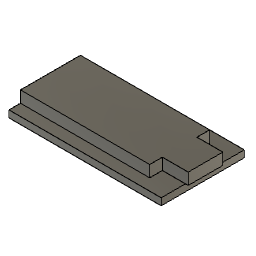
ArduinoProMicro_Pinless (Autodesk Fusion 360 design; units mm, degrees)
Autodesk Fusion 360 part; units mm, degrees
sketch "スケッチ1" plane through (0, 0, 0) normal (0, 0, 1) x (1, 0, 0)
  line L0 (0, 0) -> (33, 0)
  line L1 (33, 0) -> (33, 18)
  line L2 (33, 18) -> (0, 18)
  line L3 (0, 18) -> (0, 0)
  dimension "d1" = 33
  dimension "d2" = 18
  constraint horizontal L0
  constraint vertical L1
  constraint horizontal L2
  constraint vertical L3
  constraint coincident L0.start L3.end
  measures "d1" distance of L0.start L0.end
  measures "d2" distance of L0.start L2.end
extrude "押し出し1" add sketch "スケッチ1" along normal blind 4
sketch "スケッチ2" plane through (0, 0, 4) normal (0, 0, 1) x (-1, 0, 0)
  line L0 (0, -18) -> (0, 0)
  line L1 (0, 0) -> (-33, 0)
  line L2 (-33, 0) -> (-33, -18)
  line L3 (-33, -18) -> (0, -18)
  line L4 (-33, -18) -> (-28, -18)
  line L5 (-28, -18) -> (-28, 0)
  line L6 (-28, 0) -> (-33, 0)
  line L7 (-33, 0) -> (-33, -18)
  line L8 (-28, -12.75) -> (-33, -12.75)
  line L9 (-33, -12.75) -> (-33, -5.25)
  line L10 (-33, -5.25) -> (-28, -5.25)
  line L11 (-28, -5.25) -> (-28, -12.75)
  line L12 (-31.75, -9) -> (-34.25, -9) construction
  line L13 (-34.25, -9) -> (-31.75, -9) construction
  line L14 (0, 0) -> (-28, 0)
  line L15 (-28, 0) -> (-28, -2.5)
  line L16 (-28, -2.5) -> (0, -2.5)
  line L17 (0, -2.5) -> (0, 0)
  line L18 (0, -18) -> (-28, -18)
  line L19 (-28, -18) -> (-28, -15.5)
  line L20 (-28, -15.5) -> (0, -15.5)
  line L21 (0, -15.5) -> (0, -18)
  dimension "d5" = 5
  dimension "d6" = 18
  dimension "d7" = 5
  dimension "d8" = 7.5
  dimension "d11" = 2.5
  dimension "d12" = 2.5
  constraint horizontal L4
  constraint vertical L5
  constraint horizontal L6
  constraint vertical L7
  constraint coincident L2.end L3.start
  constraint horizontal L8
  constraint vertical L9
  constraint horizontal L10
  constraint vertical L11
  constraint horizontal L12
  constraint midpoint L9 L12
  constraint horizontal L13
  constraint midpoint L7 L13
  constraint collinear L7 L9
  constraint collinear L12 L13
  constraint horizontal L14
  constraint vertical L15
  constraint horizontal L16
  constraint vertical L17
  constraint coincident L0.end L1.start
  constraint collinear L5 L15
  constraint horizontal L18
  constraint vertical L19
  constraint horizontal L20
  constraint vertical L21
  constraint coincident L0.start L3.end
  constraint collinear L5 L19
  measures "d5" distance of L2.end L4.end
  measures "d6" distance of L2.end L1.end
  measures "d7" distance of L8.start L8.end
  measures "d8" distance of L8.start L10.end
  measures "d11" distance of L0.end L16.end
  measures "d12" distance of L0.start L20.end
extrude "押し出し2" cut sketch "スケッチ2" against normal blind 2.5 contours L0 L3 L5 L18 L19 L20 L21 | L2 L3 L4 L5 L7 L8 L19 | L0 L1 L5 L14 L15 L16 L17 | L1 L2 L5 L6 L7 L10 L15
sketch "スケッチ3" plane through (33, 0, 0) normal (1, 0, 0) x (0, 1, 0)
  line L0 (5.25, 4) -> (5.25, 1.5)
  line L1 (5.25, 1.5) -> (0, 1.5)
  line L2 (0, 1.5) -> (0, 0)
  line L3 (0, 0) -> (18, 0)
  line L4 (18, 0) -> (18, 1.5)
  line L5 (18, 1.5) -> (12.75, 1.5)
  line L6 (12.75, 1.5) -> (12.75, 4)
  line L7 (12.75, 4) -> (5.25, 4)
  line L8 (12.75, 1.5) -> (5.25, 1.5)
  line L9 (5.25, 1.5) -> (5.25, 4)
  line L10 (5.25, 4) -> (12.75, 4)
  line L11 (12.75, 4) -> (12.75, 1.5)
  constraint horizontal L8
  constraint vertical L9
  constraint horizontal L10
  constraint vertical L11
  constraint coincident L0.start L7.end
  constraint coincident L5.end L6.start
extrude "押し出し3" add sketch "スケッチ3" along normal blind 0.6 contours L0 L6 L7 L8 L9 L10 L11
